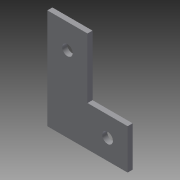
# Autodesk Inventor part: ninja
Saved by Autodesk Inventor 2013 (Build 170138000, 138)
## iProperties
Created: 2013-02-09
Part Number: ninja
Material: Generic
Document SubType Name: Modeling
Designer: Arpan
Density: 1 g/cm^3
Author: Arpan
Autodesk Inventor part; units mm, degrees
ref_plane "YZ Plane" through (0, 0, 0) normal (1, 0, 0) x (0, 1, 0)
ref_plane "XZ Plane" through (0, 0, 0) normal (0, 1, 0) x (-1, 0, 0)
ref_plane "XY Plane" through (0, 0, 0) normal (0, 0, 1) x (1, 0, 0)
sketch "Sketch1" plane through (0, 0, 0) normal (0, 0, 1) x (1, 0, 0)
  line L0 (0, 0) -> (50.8, 0)
  line L1 (50.8, 0) -> (50.8, 25.4)
  line L2 (50.8, 25.4) -> (25.4, 25.4)
  line L3 (25.4, 25.4) -> (25.4, 63.5)
  line L4 (25.4, 63.5) -> (0, 63.5)
  line L5 (0, 63.5) -> (0, 0)
  dimension "d0" = 50.8
  dimension "d2" = 25.4
  dimension "d3" = 25.4
  dimension "d4" = 38.1
  constraints: 12 end point, 3 parallel, 2 perpendicular, 1 horizontal
  measures "d0" distance of L0.start L0.end
  measures "d2" distance of L0.end L1.end
  measures "d3" distance of L1.end L2.end
  measures "d4" distance of L2.end L3.end
extrude "Extrusion1" add sketch "Sketch1" along normal blind 3.175
sketch "Sketch2" plane through (0, 0, 0) normal (0, 0, -1) x (-1, 0, 0)
  circle A0 centre (-38.1, 12.7) radius 3.3782 projected
  circle A1 centre (-12.7, 48.0173) radius 3.302 projected
  circle A2 centre (4.1663, 34.7761) radius 4.4593 projected
sketch "Sketch3" plane through (0, 0, 0) normal (0, 0, -1) x (-1, 0, 0)
  line L0 (0, 0) -> (-50.8, 0) projected
  line L1 (0, 63.5) -> (0, 0) projected
  line L2 (-25.4, 63.5) -> (0, 63.5) projected
  line L3 (-25.4, 25.4) -> (-25.4, 63.5) projected
  line L4 (-50.8, 25.4) -> (-25.4, 25.4) projected
  line L5 (-50.8, 0) -> (-50.8, 25.4) projected
  circle A0 centre (-38.1, 12.7) radius 3.3782 projected
  line L6 (-22.225, 38.6193) -> (-22.225, 32.0153) projected
  circle A1 centre (-38.1, 12.7) radius 3.3782 projected
extrude "Extrusion2" cut sketch "Sketch2" against normal blind 25.4 contours A0 | A1
body "Solid1"
